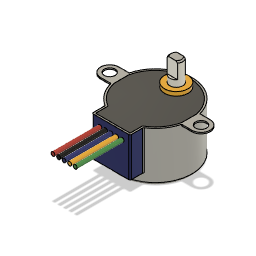
MOTOR MODEL 28BYJ-48 5V v4 (Autodesk Fusion 360 design; units mm, degrees)
Autodesk Fusion 360 part; units mm, degrees
note: some values were not read from the file. Set by a fixed rule: which sketch regions a step uses.
sketch "Sketch1" plane through (0, 0, 0) normal (0, 1, 0) x (1, 0, 0)
  circle A0 centre (0, 0) radius 14
  dimension "d1" = 28
  constraint coincident A0.centre origin
  measures "d1" diameter of A0
extrude "Extrude1" add sketch "Sketch1" along normal blind 19
sketch "Sketch2" plane through (0, 19, 0) normal (0, 1, 0) x (-1, 0, 0)
  circle A0 centre (0, 0) radius 14
  line L0 (0, 0) -> (0, -22.538) construction
  line L1 (0, 0) -> (-18.9737, 0) construction
  circle A1 centre (0, -8) radius 2.5
  dimension "d5" = 5
  dimension "d6" = 8
  constraint coincident A0.centre L0.start
  constraint vertical L0
  constraint perpendicular L0 L1
  constraint coincident L0 A1.centre
  measures "d5" diameter of A1
  measures "d6" distance of A0.centre A1.centre
extrude "Extrude2" add sketch "Sketch2" along normal blind 10 contours A1
sketch "Sketch3" plane through (0, 19, 0) normal (0, 1, 0) x (-1, 0, 0)
  circle A0 centre (0, -8) radius 2.5
  circle A1 centre (0, 0) radius 14
  circle A2 centre (0, -8) radius 4.5
  dimension "d9" = 9
  constraint concentric A0 A2
  measures "d9" diameter of A2
extrude "Extrude3" add sketch "Sketch3" along normal blind 1.5 contours A2
chamfer "Chamfer1" distance 0.5 angle 45 1 edges at (2.3308, 29, -8.904)
sketch "Sketch4" plane through (0, 29, 0) normal (0, 1, 0) x (-1, 0, 0)
  line L0 (5.7798, -15.1598) -> (-6.4865, -15.1598)
  line L1 (-6.4865, -15.1598) -> (-6.4865, -9.5)
  line L2 (-6.4865, -9.5) -> (5.7798, -9.5)
  line L3 (5.7798, -9.5) -> (5.7798, -15.1598)
  line L4 (-7.7622, -1.335) -> (6.743, -1.335)
  line L5 (6.743, -1.335) -> (6.743, -6.5)
  line L6 (6.743, -6.5) -> (-7.7622, -6.5)
  line L7 (-7.7622, -6.5) -> (-7.7622, -1.335)
  line L8 (0, -8) -> (-6.8343, -8) construction
  circle A0 centre (0, -8) radius 2
  dimension "d12" = 3
  dimension "d13" = 1.5
  constraint horizontal L0
  constraint vertical L1
  constraint horizontal L2
  constraint vertical L3
  constraint horizontal L4
  constraint vertical L5
  constraint horizontal L6
  constraint vertical L7
  constraint horizontal L8
  measures "d12" distance of L2 L6
  measures "d13" distance of L2 L8
extrude "Extrude4" cut sketch "Sketch4" against normal blind 6 contours L0 L1 L2 L3 A0 | L2 A0 | L6 A0 | L4 L5 L6 L7 A0
sketch "Sketch5" plane through (0, 19, 0) normal (0, 1, 0) x (-1, 0, 0)
  circle A0 centre (0, -8) radius 4.5
  circle A1 centre (0, 0) radius 14
  line L0 (0, 0) -> (-24.4188, 0) construction
  circle A2 centre (-17.5, 0) radius 2.1
  line L1 (-17.5, 0) -> (-17.5, 3.5) construction
  line L2 (-17.5, 3.5) -> (-13.5554, 3.5)
  arc A3 (-17.5, 3.5) -> (-17.5, -3.5) centre (-17.5, 0) ccw
  line L3 (-17.5, -3.5) -> (-13.5554, -3.5)
  line L4 (0, 0) -> (0, 16.2535) construction
  line L5 (17.5, -3.5) -> (13.5554, -3.5)
  arc A4 (17.5, -3.5) -> (17.5, 3.5) centre (17.5, 0) ccw
  line L6 (17.5, 3.5) -> (13.5554, 3.5)
  circle A5 centre (17.5, 0) radius 2.1
  dimension "d17" = 4.2
  dimension "d18" = 17.5
  dimension "d19" = 7
  constraint coincident A1.centre L0.start
  constraint horizontal L0
  constraint coincident L0 A2.centre
  constraint concentric A2 A3
  constraint coincident A2.centre L1.start
  constraint perpendicular L0 L1
  constraint parallel L0 L2
  constraint coincident A1 L2.end
  constraint symmetric L0 L1.end A3.end
  constraint symmetric L0 L2.end L3.end
  constraint perpendicular L0 L4
  constraint symmetric A2 L4 A5
  constraint symmetric L1.end L4 A4.end
  constraint symmetric L2.end L4 L6.end
  constraint symmetric A3 L4 A4
  constraint symmetric A3.end L4 L5.start
  constraint symmetric L3.end L4 L5.end
  measures "d17" diameter of A2
  measures "d18" distance of A1.centre A2.centre
  measures "d19" diameter of A3
extrude "Extrude5" add sketch "Sketch5" against normal blind 0.5 contours A1 L5 A4 L6 | A1 L2 A3 L3
sketch "Sketch6" plane through (0, 19, 0) normal (0, 1, 0) x (-1, 0, 0)
  circle A0 centre (-17.5, 0) radius 2.1
  circle A1 centre (17.5, 0) radius 2.1
  circle A2 centre (0, -8) radius 4.5
  arc A3 (13.5554, 3.5) -> (-13.5554, 3.5) centre (0, 0) ccw
  line L0 (-13.5554, 3.5) -> (-17.5, 3.5)
  arc A4 (-17.5, 3.5) -> (-17.5, -3.5) centre (-17.5, 0) ccw
  line L1 (-17.5, -3.5) -> (-13.5554, -3.5)
  arc A5 (-13.5554, -3.5) -> (13.5554, -3.5) centre (0, 0) ccw
  line L2 (13.5554, -3.5) -> (17.5, -3.5)
  arc A6 (17.5, -3.5) -> (17.5, 3.5) centre (17.5, 0) ccw
  line L3 (17.5, 3.5) -> (13.5554, 3.5)
  line L4 (7.3, 17) -> (-7.3, 17)
  line L5 (0, 0) -> (0, 20.7156) construction
  line L6 (7.3, 17) -> (7.3, 11.9461)
  line L7 (-7.3, 17) -> (-7.3, 11.9461)
  dimension "d22" = 17
  dimension "d23" = 14.6
  dimension "d24" = 7.3
  constraint horizontal L4
  constraint coincident A3.centre A5.centre
  constraint perpendicular L4 L5
  constraint perpendicular L0 L6
  constraint perpendicular L4 L7
  constraint coincident A3 L6.end
  constraint coincident A3 L7.end
  measures "d22" distance of A3.centre L4
  measures "d23" distance of L4.start L4.end
  measures "d24" horizontal distance of L4.end L5.end
extrude "Extrude6" add sketch "Sketch6" against normal blind 15 contours A3 L4 L6 L7
sketch "Sketch7" plane through (0, 19, 0) normal (0, 1, 0) x (-1, 0, 0)
  circle A0 centre (-17.5, 0) radius 2.1
  circle A1 centre (17.5, 0) radius 2.1
  circle A2 centre (0, -8) radius 4.5
  arc A3 (13.5554, 3.5) -> (7.3, 11.9461) centre (0, 0) ccw
  line L0 (7.3, 11.9461) -> (7.3, 17)
  line L1 (7.3, 17) -> (-7.3, 17)
  line L2 (-7.3, 17) -> (-7.3, 11.9461)
  arc A4 (-7.3, 11.9461) -> (-13.5554, 3.5) centre (0, 0) ccw
  line L3 (-13.5554, 3.5) -> (-17.5, 3.5)
  arc A5 (-17.5, 3.5) -> (-17.5, -3.5) centre (-17.5, 0) ccw
  line L4 (-17.5, -3.5) -> (-13.5554, -3.5)
  arc A6 (-13.5554, -3.5) -> (13.5554, -3.5) centre (0, 0) ccw
  line L5 (13.5554, -3.5) -> (17.5, -3.5)
  arc A7 (17.5, -3.5) -> (17.5, 3.5) centre (17.5, 0) ccw
  line L6 (17.5, 3.5) -> (13.5554, 3.5)
  arc A8 (17.5, -2.8) -> (17.5, 2.8) centre (17.5, 0) ccw
  line L7 (17.5, 2.8) -> (13.0019, 2.8)
  arc A9 (13.0019, 2.8) -> (6.6, 11.5469) centre (0, 0) ccw
  line L8 (6.6, 11.5469) -> (6.6, 16.3)
  line L9 (6.6, 16.3) -> (-6.6, 16.3)
  line L10 (-6.6, 16.3) -> (-6.6, 11.5469)
  arc A10 (-6.6, 11.5469) -> (-13.0019, 2.8) centre (0, 0) ccw
  line L11 (-13.0019, 2.8) -> (-17.5, 2.8)
  arc A11 (-17.5, 2.8) -> (-17.5, -2.8) centre (-17.5, 0) ccw
  line L12 (-17.5, -2.8) -> (-13.0019, -2.8)
  arc A12 (-13.0019, -2.8) -> (13.0019, -2.8) centre (0, 0) ccw
  line L13 (13.0019, -2.8) -> (17.5, -2.8)
  line L14 (13.0019, -2.8) -> (13.0019, 2.8)
  line L15 (-13.0019, -2.8) -> (-13.0019, 2.8)
  dimension "d27" = -0.7
extrude "Extrude7" cut sketch "Sketch7" against normal blind 0.01 contours A9 L8 L9 L10 A10 A12 L14 L15
fillet "Fillet1" radius 0.5 4 edges at (7.3, 11.5, 11.9461) (7.3, 11.5, 17) (-7.3, 11.5, 17) (-7.3, 11.5, 11.9461)
sketch "Sketch8" plane through (0, 0, 17) normal (0, 0, 1) x (1, 0, 0)
  line L0 (-6.8, 19) -> (-6.8, 4)
  line L1 (-6.8, 4) -> (6.8, 4)
  line L2 (6.8, 4) -> (6.8, 19)
  line L3 (6.8, 19) -> (-6.8, 19)
  line L4 (-5, 15.99) -> (5.3735, 15.99) construction
  circle A0 centre (-4.25, 15.99) radius 0.75
  line L5 (4.5, 18.99) -> (-4.5, 18.99) construction
  line L6 (0, 17.7245) -> (0, 12.8395) construction
  circle A1 centre (-2.125, 15.99) radius 0.75
  circle A2 centre (0, 15.99) radius 0.75
  circle A3 centre (2.125, 15.99) radius 0.75
  circle A4 centre (4.25, 15.99) radius 0.75
  dimension "d32" = 1.5
  dimension "d33" = 5
  dimension "d34" = 3
  dimension "d37" = 8.5
  dimension "d38" = 0
  constraint perpendicular L2 L4
  constraint coincident L4 A0.centre
  constraint perpendicular L3 L6
  constraint coincident L6 A2.centre
  measures "d32" diameter of A0
  measures "d33" distance of L4.start L6
  measures "d34" distance of L4 L5
extrude "Extrude8" add sketch "Sketch8" along normal blind 18 contours A0 | A1 | A2 | A3 | A4
fillet "Fillet2" radius 1 1 edges at (-13.0526, 0, 5.0626)
equation "d13 = d12 / 2"
equation "d18 = ( 35 / 2 ) * 1 mm"
equation "d19 = ( 3.5 * 2 ) * 1 mm"
equation "d24 = d23 / 2"
